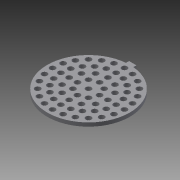
# Autodesk Inventor part: Матрица
Saved by Autodesk Inventor 2014 SP1 (Build 180222100, 222)
## iProperties
Created: 2023-07-18
Part Number: Матрица
Material: Типовые
Document SubType Name: Modeling
Designer: 1.507-7
Density: 1 g/cm^3
Appearance: По умолчанию
Author: 1.507-7
Autodesk Inventor part; units mm, degrees
ref_plane "YZ Plane" through (0, 0, 0) normal (1, 0, 0) x (0, 1, 0)
ref_plane "XZ Plane" through (0, 0, 0) normal (0, 1, 0) x (-1, 0, 0)
ref_plane "XY Plane" through (0, 0, 0) normal (0, 0, 1) x (1, 0, 0)
sketch "Эскиз1" plane through (0, 0, 0) normal (0, 0, 1) x (1, 0, 0)
  circle A0 centre (0, 0) radius 22.4
  circle A1 centre (0, 0) radius 1.5
  circle A2 centre (0, -6) radius 1.5
  circle A3 centre (0, -10.5) radius 1.5
  circle A4 centre (0, -15) radius 1.5
  circle A5 centre (0, -19.5) radius 1.5
  line L0 (-2, 21) -> (2, 21)
  line L1 (2, 21) -> (2, 24)
  line L2 (2, 24) -> (-2, 24)
  line L3 (-2, 24) -> (-2, 21)
  circle A6 centre (4.2426, -4.2426) radius 1.5
  circle A7 centre (6, 0) radius 1.5
  circle A8 centre (4.2426, 4.2426) radius 1.5
  circle A9 centre (0, 6) radius 1.5
  circle A10 centre (-4.2426, 4.2426) radius 1.5
  circle A11 centre (-6, 0) radius 1.5
  circle A12 centre (-4.2426, -4.2426) radius 1.5
  circle A13 centre (5.25, -9.0933) radius 1.5
  circle A14 centre (9.0933, -5.25) radius 1.5
  circle A15 centre (10.5, 0) radius 1.5
  circle A16 centre (9.0933, 5.25) radius 1.5
  circle A17 centre (5.25, 9.0933) radius 1.5
  circle A18 centre (0, 10.5) radius 1.5
  circle A19 centre (-5.25, 9.0933) radius 1.5
  circle A20 centre (-9.0933, 5.25) radius 1.5
  circle A21 centre (-10.5, 0) radius 1.5
  circle A22 centre (-9.0933, -5.25) radius 1.5
  circle A23 centre (-5.25, -9.0933) radius 1.5
  circle A24 centre (4.6353, -14.2658) radius 1.5
  circle A25 centre (8.8168, -12.1353) radius 1.5
  circle A26 centre (12.1353, -8.8168) radius 1.5
  circle A27 centre (14.2658, -4.6353) radius 1.5
  circle A28 centre (15, 0) radius 1.5
  circle A29 centre (14.2658, 4.6353) radius 1.5
  circle A30 centre (12.1353, 8.8168) radius 1.5
  circle A31 centre (8.8168, 12.1353) radius 1.5
  circle A32 centre (4.6353, 14.2658) radius 1.5
  circle A33 centre (0, 15) radius 1.5
  circle A34 centre (-4.6353, 14.2658) radius 1.5
  circle A35 centre (-8.8168, 12.1353) radius 1.5
  circle A36 centre (-12.1353, 8.8168) radius 1.5
  circle A37 centre (-14.2658, 4.6353) radius 1.5
  circle A38 centre (-15, 0) radius 1.5
  circle A39 centre (-14.2658, -4.6353) radius 1.5
  circle A40 centre (-12.1353, -8.8168) radius 1.5
  circle A41 centre (-8.8168, -12.1353) radius 1.5
  circle A42 centre (-4.6353, -14.2658) radius 1.5
  circle A43 centre (5.047, -18.8356) radius 1.5
  circle A44 centre (9.75, -16.8875) radius 1.5
  circle A45 centre (13.7886, -13.7886) radius 1.5
  circle A46 centre (16.8875, -9.75) radius 1.5
  circle A47 centre (18.8356, -5.047) radius 1.5
  circle A48 centre (19.5, 0) radius 1.5
  circle A49 centre (18.8356, 5.047) radius 1.5
  circle A50 centre (16.8875, 9.75) radius 1.5
  circle A51 centre (13.7886, 13.7886) radius 1.5
  circle A52 centre (9.75, 16.8875) radius 1.5
  circle A53 centre (5.047, 18.8356) radius 1.5
  circle A54 centre (0, 19.5) radius 1.5
  circle A55 centre (-5.047, 18.8356) radius 1.5
  circle A56 centre (-9.75, 16.8875) radius 1.5
  circle A57 centre (-13.7886, 13.7886) radius 1.5
  circle A58 centre (-16.8875, 9.75) radius 1.5
  circle A59 centre (-18.8356, 5.047) radius 1.5
  circle A60 centre (-19.5, 0) radius 1.5
  circle A61 centre (-18.8356, -5.047) radius 1.5
  circle A62 centre (-16.8875, -9.75) radius 1.5
  circle A63 centre (-13.7886, -13.7886) radius 1.5
  circle A64 centre (-9.75, -16.8875) radius 1.5
  circle A65 centre (-5.047, -18.8356) radius 1.5
  dimension "d1" = 3
  dimension "d2" = 3
  dimension "d3" = 3
  dimension "d4" = 3
  dimension "d5" = 3
  dimension "d6" = 4
  dimension "d7" = 3
  dimension "d10" = 360
  dimension "d14" = 360
  dimension "d18" = 360
  dimension "d22" = 360
  constraints: 66 centre point, 8 end point, 2 coincident, 2 parallel, 1 horizontal, 1 perpendicular, 132 other
  measures "d1" diameter of A1
  measures "d2" diameter of A2
  measures "d3" diameter of A3
  measures "d4" diameter of A4
  measures "d5" diameter of A5
  measures "d6" distance of L2.end L1.end
  measures "d7" distance of L1.end L0.end
extrude "Выдавливание1" add sketch "Эскиз1" along normal blind 2
